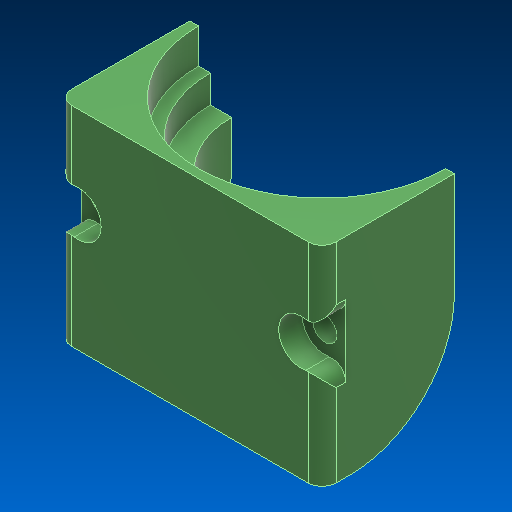
# Autodesk Inventor part: 402-gearbox-housing
Saved by Autodesk Inventor 2018 (Build 220112000, 112)
## iProperties
Created: 2020-06-11
Part Number: 402-gearbox-housing
Material: Generic
Document SubType Name: Modeling
Designer: Bunny320
Density: 1 g/cm^3
Appearance: Smooth - Dark Forest Green
Author: Bunny320
Autodesk Inventor part; units mm, degrees
ref_plane "YZ Plane" through (0, 0, 0) normal (1, 0, 0) x (0, 1, 0)
ref_plane "XZ Plane" through (0, 0, 0) normal (0, 1, 0) x (-1, 0, 0)
ref_plane "XY Plane" through (0, 0, 0) normal (0, 0, 1) x (1, 0, 0)
sketch "Sketch1" plane through (0, 0, 0) normal (0, 0, 1) x (1, 0, 0)
  line L0 (-19, -19) -> (19, -19)
  line L1 (19, -19) -> (19, 19)
  line L2 (19, 19) -> (-19, 19)
  line L3 (-19, 19) -> (-19, -19)
  line L4 (-19, -19) -> (19, 19) construction
  line L5 (19, -19) -> (-19, 19) construction
  point P0 (0, 0)
  dimension "d0" = 38
  constraints: 12 end point, 2 midpoint, 2 parallel, 2 perpendicular, 1 horizontal
  measures "d0" distance of L1.end L2.end
extrude "Extrusion1" add sketch "Sketch1" along normal blind 70
sketch "Sketch2" plane through (0, 0, 0) normal (0, 0, -1) x (-1, 0, 0)
  circle A0 centre (0, 0) radius 16.1
  dimension "d3" = 32.2
  constraints: 1 centre point, 1 coincident
  measures "d3" diameter of A0
extrude "Extrusion2" cut sketch "Sketch2" against normal blind 32
sketch "Sketch3" plane through (0, 0, 70) normal (0, 0, 1) x (1, 0, 0)
  circle A0 centre (0, 0) radius 17
  dimension "d6" = 34
  constraints: 1 centre point, 1 coincident
  measures "d6" diameter of A0
extrude "Extrusion3" cut sketch "Sketch3" against normal blind 30
sketch "Sketch4" plane through (0, 0, 40) normal (0, 0, 1) x (1, 0, 0)
  circle A0 centre (0, 0) radius 10
  dimension "d9" = 20
  constraints: 1 centre point, 1 coincident
  measures "d9" diameter of A0
extrude "Extrusion4" cut sketch "Sketch4" against normal through all
sketch "Sketch5" plane through (0, 0, 40) normal (0, 0, 1) x (1, 0, 0)
  point P0 (0, 0)
  point P1 (0, 13)
  dimension "d12" = 13
  constraints: 1 vertical alignment
  measures "d12" distance of point (0, 0) point (0, 13)
hole "Hole1" at (0, 13, 40) direction (0, 0, -1) diameter 3.4 end through all countersink diameter 7.5 countersink angle 90 clearance for "Countersunk Flat Head Hex Socket Screw DIN EN ISO 10642" size "M3" standard "DIN"
pattern_circular "Circular Pattern1" count 4 over 360 about axis through (0, 0, -10) along (0, 0, 1) of "Hole1"
sketch "Sketch7" plane through (0, 0, 0) normal (0, 1, 0) x (-1, 0, 0)
  line L0 (17, 53) -> (13, 53)
  line L1 (13, 53) -> (13, 61)
  line L2 (13, 61) -> (17, 61)
  line L3 (17, 70) -> (17, 40) projected
  line L4 (17, 61) -> (17, 53)
  line L5 (0, 45.2672) -> (0, 100.0467)
  line L6 (1.9638, 40) -> (9.8053, 40) projected
  line L7 (17, 77) -> (17, 64.9)
  line L8 (-17, 70) -> (17, 70) projected
  line L9 (17, 65) -> (16.05, 65)
  line L10 (16.05, 65) -> (16.05, 61)
  line L11 (16.05, 61) -> (17, 61)
  line L12 (17, 61) -> (17, 65)
  line L13 (17, 70) -> (17, 40) projected
  line L14 (-19, 0) -> (19, 0) projected
  point P0 (0, 0)
  point P1 (0, 0)
  dimension "d39" = 5
  dimension "d40" = 9
  dimension "d41" = 32.1
  dimension "d93" = 8
  dimension "d94" = 26
  constraints: 20 end point, 4 perpendicular, 4 point on line, 3 collinear, 2 horizontal, 1 midpoint, 1 vertical
  measures "d39" distance between parallel lines of L8 L9
  measures "d40" distance between parallel lines of L8 L11
  measures "d41" diameter of L10 L5
  measures "d93" distance of L0.end L1.end
  measures "d94" diameter of L1 L5
revolve "Revolution1" add sketch "Sketch7" angle 360 about axis through (0, 0, 45.2672) along (0, 0, 1)
sketch "Sketch8" plane through (0, 0, 70) normal (0, 0, 1) x (1, 0, 0)
  circle A0 centre (0, 0) radius 17.75
  dimension "d42" = 35.5
  constraints: 1 centre point, 1 coincident
  measures "d42" diameter of A0
extrude "Extrusion6" cut sketch "Sketch8" against normal up to surface (5 mm away)
sketch "Sketch10" plane through (-19, -19, 0) normal (0, -1, 0) x (1, 0, 0)
  line L0 (35, 81.8891) -> (3, 81.8891)
  line L1 (3, 81.8891) -> (3, 57)
  line L2 (3, 57) -> (35, 57)
  line L3 (35, 57) -> (35, 81.8891)
  line L4 (0, 0) -> (0, 70) projected
  line L5 (38, 0) -> (38, 70) projected
  line L6 (6, 61) -> (32, 61) projected
  point P0 (19, 0)
  dimension "d58" = 3
  dimension "d59" = 3
  dimension "d95" = 4
  constraints: 8 end point, 2 coincident, 2 parallel, 1 horizontal, 1 perpendicular
  measures "d58" distance between parallel lines of L4 L1
  measures "d59" distance between parallel lines of L5 L3
  measures "d95" distance between parallel lines of L6 L2
hole "Hole3" at (16, -19, 57) at (-16, -19, 57) direction (0, 1, 0) diameter 3.4 end through all counterbore diameter 6.5 counterbore depth 3.4 clearance for "Socket Head Cap Screw DIN EN ISO 4762" size "M3" standard "DIN"
sketch "Sketch11" plane through (0, 0, 70) normal (0, 0, 1) x (1, 0, 0)
  line L0 (19, 19) -> (-19, 19) projected
  line L1 (19, -19) -> (19, 19) projected
  line L2 (-19, 19) -> (19, 19)
  line L3 (19, 19) -> (19, 0)
  line L4 (19, 0) -> (-19, 0)
  line L5 (-19, 0) -> (-19, 19)
  point P0 (0, 0)
  constraints: 8 end point, 2 parallel, 1 horizontal, 1 midpoint, 1 perpendicular
extrude "Extrusion7" cut sketch "Sketch11" against normal up to surface (30 mm away)
sketch "Sketch13" plane through (0, 0, 0) normal (0, 0, -1) x (-1, 0, 0)
  line L0 (-23.6074, 22.2349) -> (23.2414, 22.2349)
  line L1 (23.2414, 22.2349) -> (23.2414, -22.6009)
  line L2 (23.2414, -22.6009) -> (-23.6074, -22.6009)
  line L3 (-23.6074, -22.6009) -> (-23.6074, 22.2349)
  point P0 (0, 0)
  constraints: 8 end point, 2 parallel, 1 horizontal, 1 perpendicular
extrude "Extrusion8" cut sketch "Sketch13" against normal up to surface (40 mm away)
fillet "Fillet2" radius 15 2 edges at (-18, 0, 40) (18, 0, 40)
fillet "Fillet3" radius 2 8 edges at (-19, -19, 64.125) (19, -19, 64.125) (19, -19, 47.875) (-19, -19, 47.875) (-19, -17.3, 58.25) (-19, -17.3, 55.75) (19, -17.3, 58.25) (19, -17.3, 55.75)
sketch "Sketch6" plane through (0, 0, 0) normal (0, 1, 0) x (-1, 0, 0)
  line L0 (-59.915, -50.2576) -> (49.2575, -50.2576)
  line L1 (49.2575, -50.2576) -> (49.2575, 450.4062)
  line L2 (49.2575, 450.4062) -> (-59.915, 450.4062)
  line L3 (-59.915, 450.4062) -> (-59.915, -50.2576)
  point P0 (0, 0)
  constraints: 8 end point, 2 parallel, 1 horizontal, 1 perpendicular
equation "\"d41\" = bearing_61705_outer"
equation "\"d59\" = d58"
equation "\"bearing_61807_inner\" = 35"
equation "\"bearing_61807_outer\" = 47.1"
equation "\"bearing_61814_outer\" = 90.1"
equation "\"bearing_61705_outer\" = 32.1"
equation "\"bearing_61705_inner\" = 25"
equation "\"M3_adjustable\" = 3.2"
equation "\"bearing_606_outer\" = 17.1"
equation "\"gearbox_35_outer\" = 32.3"
body "Solid1"
